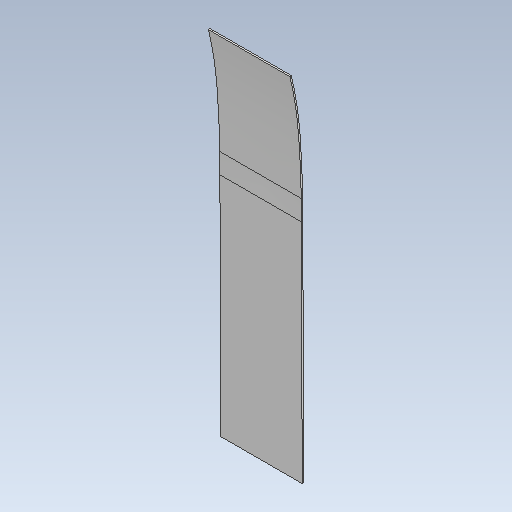
# Autodesk Inventor part: bottom_offset_plate
Saved by Autodesk Inventor 2020.3 (Build 243373010, 373A)
## iProperties
Created: 2021-01-30
Part Number: bottom_offset_plate
Material: Generic
Document SubType Name: Modeling
Designer: kardo
Density: 1 g/cm^3
Appearance: Default
Mass: 25.5972 g
Surface Area: 435.652 cm^2
Volume: 25.5972 cm^3
Author: kardo
Autodesk Inventor part; units mm, degrees
ref_plane "XZ Plane" through (0, 0, 0) normal (0, 1, 0) x (-1, 0, 0)
derived "bottom_offset_wall.ipt"
sketch "profile" plane through (0, 0, 0) normal (1, 0, 0) x (0, 1, 0)
  line L0 (-102, 16.8245) -> (-102, 5.6919) construction
  line L1 (-204, 9.5169) -> (-204, 14.025) construction
  line L2 (0, 19.935) -> (0, 0) construction
  line L3 (56.1, 3.9229) -> (56.1, 21.6458) construction
  line L4 (112.2, 7.8458) -> (112.2, 23.3566) construction
  line L5 (-193.8, 14.025) -> (112.2, 23.3566)
  line L6 (17.2125, 13.5685) -> (112.2, 16.4652) construction
  line L7 (-193.8, 14.025) -> (0, 13.529) construction
  line L8 (-193.8, 14.025) -> (-193.8, 12.825)
  line L9 (-193.8, 12.825) -> (0, 13.529)
  spline S0 degree 4 poles (0, 13.529) (2.1516, 13.5235) (6.4547, 13.5125) (10.7595, 13.3717) (15.0615, 13.5029) (17.2125, 13.5685) knots 0 0 0 0 0 0.5 1 1 1 1 1
  spline S1 degree 3 poles (17.2125, 13.5685) (49.0693, 14.54) (80.9261, 15.5115) (112.2, 23.3566) knots 0 0 0 0 1 1 1 1
derived "base_sketch.ipt"
sketch "bulkhead_main" plane through (0, 0, 0) normal (0, 1, 0) x (-1, 0, 0)
  line L0 (0, 19.935) -> (28.764, 19.935)
  line L1 (28.764, 19.935) -> (28.764, 13.529)
  line L2 (28.764, 13.529) -> (62.322, 13.529)
  line L3 (0, 0) -> (-11.5056, 0)
  line L4 (-11.5056, 0) -> (-11.5056, -2.4868)
  line L5 (-11.5056, -2.4868) -> (-34.5168, -2.4868)
  line L6 (-34.5168, -2.4868) -> (-57.528, 27.54)
  line L7 (19.176, 46.818) -> (62.322, 46.818)
  line L8 (0, 19.935) -> (0, 0)
  line L9 (86.7165, 0) -> (-84.045, 0)
  line L10 (0, -13.6228) -> (0, 64.3297)
  line L11 (62.322, 46.818) -> (62.322, 13.529)
  line L12 (0, 35.7) -> (-57.528, 27.54) construction
  line L13 (-11.5056, -2.4868) -> (0, -2.4868) construction
  line L14 (0, -2.4868) -> (0, 0) construction
  spline S0 degree 4 poles (-57.528, 27.54) (-46.0483, 34.2051) (-30.6129, 40.5281) (-11.2214, 45.0414) (8.3201, 46.818) (15.5662, 46.818) (19.176, 46.818) knots 0 0 0 0 0 0.630279 0.815816 1 1 1 1 1
  point P0 (0, 45.9)
  point P1 (-38.352, 36.72)
  point P2 (-19.176, 42.5952)
  point P3 (0, 13.529)
ref_plane "Work Plane1" through (0, -193.8, 12.825) normal (0, 0.9999934, 0.0036326) x (-1, 0, 0)
sketch "Sketch4" plane through (0, -193.8, 12.825) normal (0, 0.9999934, 0.0036326) x (-1, 0, 0)
  line L0 (28.764, 0) -> (62.322, 0) projected
  line L1 (62.322, 0) -> (97.08, 0)
  line L2 (27.564, -1.2) -> (97.08, -1.2)
  line L3 (97.08, -1.2) -> (97.08, 0)
  line L4 (28.764, 0) -> (27.564, 0)
  line L5 (27.564, 0) -> (27.564, -1.2)
  point P0 (0, -13.5289)
  point P1 (0, 0)
  dimension "d4" = 1.2
  dimension "d5" = 1.2
  dimension "d6" = 34.758
  dimension "d7" = 34.758
  constraints: 10 end point, 2 collinear, 2 perpendicular, 1 parallel
  measures "d4" distance between parallel lines of L2 L1
  measures "d5" distance of L0.start L4.end
  measures "d6" distance of L0.end L4.end
  measures "d7" distance of L0.end L1.end
ref_plane "Work Plane2" through (-27.564, -193.8, 12.825) normal (1, 0, 0) x (0, 1, 0)
sketch "Sketch5" plane through (-27.564, -193.8, 12.825) normal (1, 0, 0) x (0, 1, 0)
  line L0 (0, 0) -> (193.8, 0.704) projected
  spline S0 degree 4 poles (193.8, 0.704) (195.9516, 0.6985) (200.2547, 0.6875) (204.5595, 0.5467) (208.8615, 0.6779) (211.0125, 0.7435) knots 0 0 0 0 0 0.5 1 1 1 1 1 projected
  spline S1 degree 3 poles (211.0125, 0.7435) (242.8693, 1.715) (274.7261, 2.6865) (306, 10.5316) knots 0 0 0 0 1 1 1 1 projected
  point P0 (193.8, -12.825)
  point P1 (308, 10.5926)
sweep "Sweep1" add profiles "Sketch4" path "Sketch5"
equation "\"d4\" = decking_thickness"
equation "\"d5\" = decking_thickness"
equation "\"d7\" = d6"
equation "\"decking_thickness\" = 1.2"
body "Solid1"
